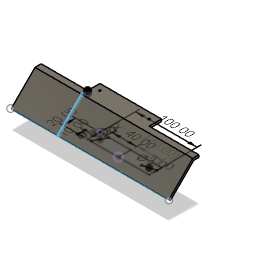
Main (Components all together) v50 (Autodesk Fusion 360 archive; units mm, degrees)
design "Front Shield"
Autodesk Fusion 360 part; units mm, degrees
sketch "Attacher" plane through (0, 0, 0) normal (0, 1, 0) x (1, 0, 0)
  line L0 (0, 0) -> (100, 0)
  line L1 (100, 0) -> (100, -20)
  line L2 (100, -20) -> (0, -20)
  line L3 (0, -20) -> (0, 0)
  circle A0 centre (10, -10) radius 1.5
  line L4 (50, -20) -> (50, 0)
  circle A1 centre (90, -10) radius 1.5
  point P0 (90, -10)
  dimension "d1" = 100
  dimension "d2" = 20
  dimension "d3" = 3
  dimension "d4" = 40
  dimension "d5" = 3
  dimension "d6" = 40
  dimension "d7" = 10
  constraint horizontal L0
  constraint vertical L1
  constraint horizontal L2
  constraint vertical L3
  constraint coincident L0.start L3.end
  constraint midpoint L2 L4.start
  constraint midpoint L0 L4.end
  constraint symmetric A0.centre L4 P0
  constraint coincident P0 A1.centre
  measures "d1" distance of L1.end L2.end
  measures "d2" distance of L0.start L2.end
  measures "d3" diameter of A0
  measures "d4" distance of A0.centre L4
  measures "d5" diameter of A1
  measures "d6" distance of L4 P0
  measures "d7" distance of L2 A0.centre
extrude "Extrude1" add sketch "Attacher" along normal blind 3.5 contours L0 L2 L3 L4 makes body 1
extrude "Extrude2" add sketch "Attacher" along normal blind 3.5 contours L0 L1 L2 L4 bodies 1
move_body "Move1" bodies 1 to x (1, 0, 0) y (0, 1, 0) z (0, 0, 1) at (0, 15, 0)
move_body "Move2" bodies 1 to x (1, 0, 0) y (0, 1, 0) z (0, 0, 1) at (0, 50, 0)
sketch "FrontShield" plane through (0, 0, 0) normal (1, 0, 0) x (0, 0, -1)
  line L0 (-20, 68.5) -> (-30, 68.5)
  line L1 (-30, 68.5) -> (-68.8909, 29.6091)
  line L2 (-68.8909, 29.6091) -> (-66.416, 27.1343)
  line L3 (-66.416, 27.1343) -> (-28.5503, 65)
  line L4 (-28.5503, 65) -> (-20, 65)
  line L5 (-20, 68.5) -> (-20, 65)
  line L6 (-66.416, 27.1343, 0) -> (-66.416, 27.1343, 100)
  line L7 (-66.416, 27.1343, 0) -> (-66.416, 27.1343, -78.5)
  line L8 (-66.416, 27.1343, 100) -> (-66.416, 27.1343, 178.5)
  point P0 (-20, 68.5)
  point P1 (-20, 65)
  point P2 (-20, 0)
  dimension "d12" = 10
  dimension "d14" = 135
  dimension "d15" = 3.5
  dimension "d18" = 55
  dimension "d24" = 100
  dimension "d25" = 78.5
  dimension "d26" = 78.5
  constraint coincident P0 L0.start
  constraint perpendicular L1 L2
  constraint perpendicular L2 L3
  constraint coincident P1 L4.end
  constraint parallel L0 L4
  constraint perpendicular L4 L5
  measures "d12" distance of P0 L0.end
  measures "d14" angle of L0 L1
  measures "d15" distance of L1.end L2.end
  measures "d18" distance of L0.end L1.end
  measures "d24" distance of L2.end L3.start
  measures "d25" distance of L2.end L3.start
  measures "d26" distance of L2.end L3.start
extrude "Extrude5" add sketch "FrontShield" along normal blind 150 bodies 1
extrude "Extrude6" add sketch "FrontShield" against normal blind 50 bodies 1
copy_body "Body->Comp1" bodies 1 removing the originals makes body 2 in component "Shield"
extrude "Extrude1'" add 1 faces at (-50, 54.3697, 42.4804) along direction (-1, 0, 0) blind 25 on bodies 2 bodies 2 in component "Shield"
extrude "Extrude2'" add 1 faces at (150, 54.3697, 42.4804) along direction (1, 0, 0) blind 25 on bodies 2 bodies 2 in component "Shield"
extrude "Extrude3" add 1 faces at (-75, 54.3697, 42.4804) along direction (-1, 0, 0) blind 3.5 on bodies 2 bodies 2 in component "Shield"
extrude "Extrude4" add 1 faces at (175, 54.3697, 42.4804) along direction (1, 0, 0) blind 3.5 on bodies 2 bodies 2 in component "Shield"
extrude "Extrude5'" cut 1 faces at (178.5, 54.3697, 42.4804) along direction (-1, 0, 0) blind 2.45 on bodies 2 bodies 2 in component "Shield"
extrude "Extrude6'" cut 1 faces at (-78.5, 54.3697, 42.4804) along direction (1, 0, 0) blind 2.45 on bodies 2 bodies 2 in component "Shield"
extrude "Extrude7" add 1 faces at (176.05, 54.3697, 42.4804) along direction (1, 0, 0) blind 2.45 on bodies 2 bodies 2 in component "Shield"
extrude "Extrude8" add 1 faces at (178.5, 54.3697, 42.4804) along direction (1, 0, 0) blind 1.5 on bodies 2 bodies 2 in component "Shield"
fillet "Fillet1" radius 4 1 edges at (180, 28.3717, 67.6534) on bodies 2 in component "Shield"
fillet "Fillet2" radius 4 1 edges at (-76.05, 28.3717, 67.6534) on bodies 2 in component "Shield"
delete_face "DeleteFace1" 1 faces at (178.8949, 28.8358, 66.3644) on bodies 2 in component "Shield"
extrude "Extrude9" cut 1 faces at (180, 54.3697, 42.4804) along direction (-1, 0, 0) blind 10.67 on bodies 2 bodies 2 in component "Shield"
delete_face "DeleteFace2" 1 faces at (-76.0319, 30.5188, 64.6814) on bodies 2 in component "Shield"
extrude "Extrude10" cut 1 faces at (-76.05, 54.3697, 42.4804) along direction (1, 0, 0) blind 0.682 on bodies 2 bodies 2 in component "Shield"
extrude "Extrude11" add 1 faces at (169.33, 54.3697, 42.4804) along direction (1, 0, 0) blind 11.408 on bodies 2 bodies 2 in component "Shield"
extrude "Extrude3'" [suppressed]
extrude "Extrude4'" [suppressed]
component "Shield" placed x (1, 0, 0) y (0, 1, 0) z (0, 0, 1) at (0, 0, 0)
equation "d4 = d6"

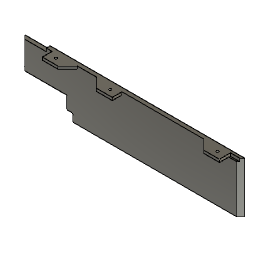
design "Side Wall"
Autodesk Fusion 360 part; units mm, degrees
sketch "Sketch1" plane through (0, 0, 0) normal (0, 0, 1) x (1, 0, 0)
  line L0 (-92.95, 30) -> (190, 30)
  line L1 (190, 30) -> (190, 25)
  line L2 (190, 25) -> (-92.95, 25)
  line L3 (-92.95, 25) -> (-92.95, 30)
  circle A0 centre (-42.95, 20) radius 1.5
  circle A1 centre (27.05, 20) radius 1.5
  circle A2 centre (165, 20) radius 1.5
  line L4 (-52.95, 25) -> (-32.95, 25)
  line L5 (-32.95, 25) -> (-32.95, 12.5)
  line L6 (-32.95, 12.5) -> (-52.95, 12.5)
  line L7 (-52.95, 12.5) -> (-52.95, 25)
  line L8 (17.05, 25) -> (37.05, 25)
  line L9 (37.05, 25) -> (37.05, 12.5)
  line L10 (37.05, 12.5) -> (17.05, 12.5)
  line L11 (17.05, 12.5) -> (17.05, 25)
  line L12 (155, 25) -> (175, 25)
  line L13 (175, 25) -> (175, 12.5)
  line L14 (175, 12.5) -> (155, 12.5)
  line L15 (155, 12.5) -> (155, 25)
  line L16 (-92.95, 30) -> (-87.95, 25)
  line L17 (190, 30) -> (185, 25)
  line L18 (-32.95, 12.5) -> (-20.45, 25)
  line L19 (17.05, 12.5) -> (4.55, 25)
  line L20 (155, 12.5) -> (142.5, 25)
  dimension "d1" = 282.95
  dimension "d2" = 5
  dimension "d3" = 3
  dimension "d4" = 10
  dimension "d5" = 50
  dimension "d6" = 3
  dimension "d7" = 70
  dimension "d8" = 10
  dimension "d9" = 3
  dimension "d10" = 25
  dimension "d11" = 10
  dimension "d12" = 10
  dimension "d13" = 10
  dimension "d14" = 7.5
  dimension "d15" = 10
  dimension "d16" = 7.5
  dimension "d17" = 10
  dimension "d18" = 10
  dimension "d19" = 10
  dimension "d20" = 7.5
  dimension "d21" = 45
  dimension "d22" = 45
  dimension "d24" = 45
  dimension "d25" = 45
  dimension "d27" = 45
  dimension "d36" = 40
  constraint horizontal L0
  constraint vertical L1
  constraint horizontal L2
  constraint vertical L3
  constraint horizontal L4
  constraint vertical L5
  constraint horizontal L6
  constraint vertical L7
  constraint coincident L2 L4.start
  constraint horizontal L8
  constraint vertical L9
  constraint horizontal L10
  constraint vertical L11
  constraint coincident L2 L8.start
  constraint horizontal L12
  constraint vertical L13
  constraint horizontal L14
  constraint vertical L15
  constraint coincident L2 L12.start
  constraint coincident L2 L16.end
  constraint coincident L2 L17.end
  constraint coincident L2 L18.end
  constraint coincident L2 L19.end
  constraint coincident L2 L20.end
  measures "d1" distance of L1 L3
  measures "d2" distance of L0.start L2.end
  measures "d3" diameter of A0
  measures "d4" distance of L0 A0.centre
  measures "d5" distance of L3 A0.centre
  measures "d6" diameter of A1
  measures "d7" distance of A0.centre A1.centre
  measures "d8" distance of L0 A1.centre
  measures "d9" diameter of A2
  measures "d10" distance of L1 A2.centre
  measures "d11" distance of L0 A2.centre
  measures "d12" distance of A0.centre L7
  measures "d13" distance of A0.centre L5
  measures "d14" distance of A0.centre L6
  measures "d15" distance of A1.centre L11
  measures "d16" distance of A1.centre L10
  measures "d17" distance of A1.centre L9
  measures "d18" distance of A2.centre L15
  measures "d19" distance of A2.centre L13
  measures "d20" distance of A2.centre L14
  measures "d21" angle of L3 L16
  measures "d22" angle of L1 L17
  measures "d24" angle of L5 L18
  measures "d25" angle of L11 L19
  measures "d27" angle of L15 L20
  measures "d36" distance of L2.end L4.start
extrude "Extrude8" add sketch "Sketch1" against normal blind 3.5 contours L0 L2 L4 L8 L12 L16 L17 | L2 L4 L5 L6 L7 | L2 L12 L13 L14 L15 | L2 L5 L18 | L2 L15 L20 | L2 L11 L19 | L2 L8 L9 L10 L11
extrude "Extrude9" add sketch "Sketch1" against normal blind 65.5 contours L0 L2 L4 L8 L12 L16 L17
sketch "Sketch5" plane through (0, 0, 0) normal (0, 0, 1) x (1, 0, 0)
  line L0 (-92.95, 30) -> (-60.45, 30)
  line L1 (-60.45, 30) -> (-60.45, 25)
  line L2 (-60.45, 25) -> (-92.95, 25)
  line L3 (-92.95, 25) -> (-92.95, 30)
  line L4 (-92.95, 25) -> (-92.95, 30)
  line L5 (190, 30) -> (190, 25)
  line L6 (-92.95, 30) -> (190, 30)
  line L7 (190, 25) -> (175, 25)
  line L8 (175, 25) -> (175, 26.8)
  line L9 (175, 26.8) -> (190, 26.8)
  line L10 (190, 26.8) -> (190, 25)
  dimension "d54" = 250.45
  dimension "d55" = 32.5
  dimension "d56" = 5
  dimension "d64" = 1.8
  dimension "d65" = 15
  constraint horizontal L0
  constraint vertical L1
  constraint horizontal L2
  constraint vertical L3
  constraint horizontal L7
  constraint vertical L8
  constraint horizontal L9
  constraint vertical L10
  constraint coincident L5.end L7.start
  measures "d54" distance of L1 L5
  measures "d55" distance of L1 L3
  measures "d56" distance of L2 L6
  measures "d64" distance of L7 L9
  measures "d65" distance of L8 L10
extrude "Extrude10" cut sketch "Sketch5" against normal blind 4 contours L0 L1 L2 L3 L4 L6
sketch "Sketch7" plane through (0, 0, -65.5) normal (0, 0, -1) x (1, 0, 0)
  line L0 (-87.95, -25) -> (-92.95, -30)
  line L1 (-92.95, -30) -> (190, -30)
  line L2 (190, -30) -> (185, -25)
  line L3 (185, -25) -> (-87.95, -25)
  line L4 (-92.95, -30) -> (-34.15, -30)
  line L5 (-34.15, -30) -> (-34.15, -25)
  line L6 (-34.15, -25) -> (-92.95, -25)
  line L7 (-92.95, -25) -> (-92.95, -30)
  line L8 (-34.15, -30) -> (-26.15, -30)
  line L9 (-26.15, -30) -> (-26.15, -25)
  line L10 (-26.15, -25) -> (-34.15, -25)
  line L11 (-34.15, -25) -> (-34.15, -30)
  dimension "d60" = 5
  dimension "d61" = 58.8
  dimension "d68" = 8
  constraint horizontal L4
  constraint vertical L5
  constraint horizontal L6
  constraint vertical L7
  constraint coincident L3 L5.end
  constraint coincident L0.end L1.start
  constraint horizontal L8
  constraint vertical L9
  constraint horizontal L10
  constraint vertical L11
  constraint coincident L3 L9.end
  measures "d60" distance of L4 L6
  measures "d61" distance of L5 L7
  measures "d68" distance of L9 L11
extrude "Extrude11" cut sketch "Sketch7" against normal blind 26.25 contours L0 L1 L3 L4 L5 L6 L11
extrude "Extrude12" cut sketch "Sketch5" against normal blind 4 contours L5 L7 L8 L9 L10
extrude "Extrude13" cut sketch "Sketch7" against normal blind 10 contours L1 L3 L5 L8 L9 L10 L11
fillet "Fillet1" radius 2 1 edges at (-26.15, 27.5, -55.5)

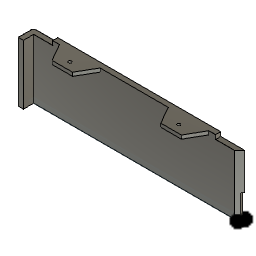
design "Front Wall"
Autodesk Fusion 360 part; units mm, degrees
sketch "Sketch1" plane through (0, 0, 0) normal (0, 0, 1) x (1, 0, 0)
  line L0 (-156.1, 40) -> (50, 40)
  line L1 (50, 40) -> (50, 35)
  line L2 (50, 35) -> (-156.1, 35)
  line L3 (-156.1, 35) -> (-156.1, 40)
  circle A0 centre (-106.1, 25.5) radius 1.5
  circle A1 centre (0, 25.5) radius 1.5
  line L4 (-116.1, 35) -> (-96.1, 35)
  line L5 (-96.1, 35) -> (-96.1, 18)
  line L6 (-96.1, 18) -> (-116.1, 18)
  line L7 (-116.1, 18) -> (-116.1, 35)
  line L8 (-10, 35) -> (10, 35)
  line L9 (10, 35) -> (10, 18)
  line L10 (10, 18) -> (-10, 18)
  line L11 (-10, 18) -> (-10, 35)
  line L12 (-96.1, 18) -> (-86.285, 35)
  line L13 (-116.1, 18) -> (-125.915, 35)
  line L14 (-10, 18) -> (-19.815, 35)
  line L15 (10, 18) -> (19.815, 35)
  line L16 (50, 40) -> (45, 35)
  dimension "d1" = 206.1
  dimension "d2" = 5
  dimension "d3" = 3
  dimension "d4" = 3
  dimension "d5" = 50
  dimension "d6" = 14.5
  dimension "d7" = 50
  dimension "d8" = 14.5
  dimension "d9" = 10
  dimension "d10" = 10
  dimension "d11" = 7.5
  dimension "d12" = 10
  dimension "d13" = 10
  dimension "d14" = 7.5
  dimension "d15" = 30
  dimension "d16" = 30
  dimension "d17" = 30
  dimension "d18" = 30
  dimension "d19" = 45
  constraint horizontal L0
  constraint vertical L1
  constraint horizontal L2
  constraint vertical L3
  constraint horizontal L4
  constraint vertical L5
  constraint horizontal L6
  constraint vertical L7
  constraint coincident L2 L4.start
  constraint horizontal L8
  constraint vertical L9
  constraint horizontal L10
  constraint vertical L11
  constraint coincident L2 L8.start
  constraint coincident L2 L12.end
  constraint coincident L2 L13.end
  constraint coincident L2 L14.end
  constraint coincident L2 L15.end
  constraint coincident L2 L16.end
  measures "d1" distance of L1 L3
  measures "d2" distance of L0.start L2.end
  measures "d3" diameter of A0
  measures "d4" diameter of A1
  measures "d5" distance of L3 A0.centre
  measures "d6" distance of L0 A0.centre
  measures "d7" distance of L1 A1.centre
  measures "d8" distance of L0 A1.centre
  measures "d9" distance of A1.centre L11
  measures "d10" distance of A1.centre L9
  measures "d11" distance of A1.centre L10
  measures "d12" distance of A0.centre L5
  measures "d13" distance of A0.centre L7
  measures "d14" distance of A0.centre L6
  measures "d15" angle of L7 L13
  measures "d16" angle of L5 L12
  measures "d17" angle of L11 L14
  measures "d18" angle of L9 L15
  measures "d19" angle of L1 L16
extrude "Extrude1" add sketch "Sketch1" against normal blind 3.5 contours L2 L7 L13 | L2 L9 L15 | L2 L4 L5 L6 L7 | L2 L8 L9 L10 L11 | L2 L5 L12 | L2 L11 L14 makes body 1 at (-95.6839, 26.314, 0) makes body 2 at (10.4161, 26.314, 0)
extrude "Extrude2" add sketch "Sketch1" against normal blind 62.2 contours L0 L2 L3 L4 L8 L16 bodies 1 2
sketch "Sketch3" plane through (0, 0, 0) normal (0, 0, 1) x (-1, 0, 0)
  circle A0 centre (0, -25.5) radius 1.5
  circle A1 centre (106.1, -25.5) radius 1.5
  line L0 (96.1, -18) -> (86.285, -35)
  line L1 (86.285, -35) -> (19.815, -35)
  line L2 (19.815, -35) -> (10, -18)
  line L3 (10, -18) -> (-10, -18)
  line L4 (-10, -18) -> (-19.815, -35)
  line L5 (-19.815, -35) -> (-45, -35)
  line L6 (-45, -35) -> (-50, -40)
  line L7 (-50, -40) -> (156.1, -40)
  line L8 (125.915, -35) -> (116.1, -18)
  line L9 (116.1, -18) -> (96.1, -18)
  line L10 (-50, -40) -> (-26.5, -40)
  line L11 (-26.5, -40) -> (-26.5, -35)
  line L12 (-26.5, -35) -> (-50, -35)
  line L13 (-50, -35) -> (-50, -40)
  line L14 (156.1, -40) -> (132.6, -40)
  line L15 (132.6, -40) -> (132.6, -35)
  line L16 (132.6, -35) -> (156.1, -35)
  line L17 (156.1, -35) -> (156.1, -40)
  line L18 (156.1, -40) -> (156.1, -35)
  line L19 (156.1, -35) -> (125.915, -35)
  dimension "d28" = 5
  dimension "d29" = 23.5
  dimension "d30" = 5
  dimension "d31" = 23.5
  constraint horizontal L10
  constraint vertical L11
  constraint horizontal L12
  constraint vertical L13
  constraint coincident L5 L11.end
  constraint coincident L6.end L7.start
  constraint horizontal L14
  constraint vertical L15
  constraint horizontal L16
  constraint vertical L17
  constraint coincident L7.end L14.start
  measures "d28" distance of L7.end L16.end
  measures "d29" distance of L15 L17
  measures "d30" distance of L10 L12
  measures "d31" distance of L11 L13
extrude "Extrude3" cut sketch "Sketch3" against normal blind 4 contours L7 L14 L15 L16 L17 L18 L19 | L5 L6 L7 L10 L11 L12 bodies 1
sketch "Sketch4" plane through (0, 0, -62.2) normal (0, 0, -1) x (1, 0, 0)
  line L0 (45, -35) -> (-156.1, -35)
  line L1 (-156.1, -35) -> (-156.1, -40)
  line L2 (-156.1, -40) -> (50, -40)
  line L3 (50, -40) -> (45, -35)
  line L4 (50, -40) -> (48, -40)
  line L5 (48, -40) -> (48, -35)
  line L6 (48, -35) -> (50, -35)
  line L7 (50, -35) -> (50, -40)
  dimension "d34" = 5
  dimension "d35" = 2
  constraint horizontal L4
  constraint vertical L5
  constraint horizontal L6
  constraint vertical L7
  constraint coincident L0 L5.end
  constraint coincident L2.end L3.start
  measures "d34" distance of L4 L6
  measures "d35" distance of L5 L7
extrude "Extrude5" cut sketch "Sketch4" against normal blind 22.4 contours L2 L3 L4 L5 bodies 1
sketch "Sketch5" plane through (0, 35, 0) normal (0, -1, 0) x (1, 0, 0)
  line L0 (-132.6, -4) -> (-156.1, -4)
  line L1 (-156.1, -4) -> (-156.1, -62.2)
  line L2 (-156.1, -62.2) -> (45, -62.2)
  line L3 (45, -62.2) -> (45, -4)
  line L4 (45, -4) -> (26.5, -4)
  line L5 (26.5, -4) -> (26.5, 0)
  line L6 (26.5, 0) -> (19.815, 0)
  line L7 (19.815, 0) -> (19.815, -3.5)
  line L8 (19.815, -3.5) -> (-19.815, -3.5)
  line L9 (-19.815, -3.5) -> (-19.815, 0)
  line L10 (-19.815, 0) -> (-86.285, 0)
  line L11 (-86.285, 0) -> (-86.285, -3.5)
  line L12 (-86.285, -3.5) -> (-125.915, -3.5)
  line L13 (-125.915, -3.5) -> (-125.915, 0)
  line L14 (-125.915, 0) -> (-132.6, 0)
  line L15 (-132.6, 0) -> (-132.6, -4)
  line L16 (-156.1, -4) -> (-151.1, -4)
  line L17 (-151.1, -4) -> (-151.1, -62.2)
  line L18 (-151.1, -62.2) -> (-156.1, -62.2)
  line L19 (-156.1, -62.2) -> (-156.1, -4)
  dimension "d40" = 5
  constraint horizontal L16
  constraint vertical L17
  constraint horizontal L18
  constraint vertical L19
  constraint coincident L2 L17.end
  constraint coincident L0.end L1.start
  measures "d40" distance of L17 L19
extrude "Extrude6" add sketch "Sketch5" along normal blind 10 contours L0 L1 L2 L16 L17 L18 L19 bodies 1
fillet "Fillet1" radius 2 1 edges at (-156.1, 40, -33.1) on bodies 1
